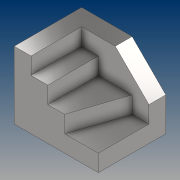
# Autodesk Inventor part: 15
Saved by Autodesk Inventor 2020.2 (Build 242310000, 310)
## iProperties
Created: 2020-09-17
Part Number: 15
Material: 鋼、碳鋼
Document SubType Name: Modeling
Designer: user
Density: 7.85 g/cm^3
Appearance: 半拋光
Mass: 412.125 g
Surface Area: 105.991 cm^2
Volume: 52.5 cm^3
Author: user
Autodesk Inventor part; units mm, degrees
ref_plane "YZ Plane" through (0, 0, 0) normal (1, 0, 0) x (0, 1, 0)
ref_plane "XZ Plane" through (0, 0, 0) normal (0, 1, 0) x (-1, 0, 0)
ref_plane "XY Plane" through (0, 0, 0) normal (0, 0, 1) x (1, 0, 0)
sketch "草圖1" plane through (0, 0, 0) normal (0, 1, 0) x (-1, 0, 0)
  line L0 (0, 0) -> (-50, 0)
  line L1 (-50, 0) -> (-50, -40)
  line L2 (-50, -40) -> (0, -40)
  line L3 (0, -40) -> (0, 0)
  dimension "d0" = 50
  dimension "d1" = 40
  constraints: 8 end point, 2 parallel, 1 horizontal, 1 perpendicular
  measures "d0" distance of L0.start L0.end
  measures "d1" distance of L2.end L0.start
extrude "擠出1" add sketch "草圖1" along normal blind 40
sketch "草圖2" plane through (0, 0, 0) normal (0, 0, 1) x (1, 0, 0)
  line L0 (0, 0) -> (0, 40) projected
  line L1 (0, 40) -> (50, 40) projected
  line L2 (50, 40) -> (50, 0) projected
  line L3 (50, 0) -> (0, 0) projected
  line L4 (0, 40) -> (50, 40) projected
  line L5 (10, 40) -> (10, 30)
  line L6 (10, 30) -> (20, 30)
  line L7 (20, 30) -> (20, 20)
  line L8 (20, 20) -> (40, 20)
  line L9 (40, 20) -> (40, 10)
  line L10 (40, 10) -> (50, 10)
  dimension "d4" = 10
  dimension "d5" = 20
  dimension "d6" = 30
  dimension "d7" = 10
  dimension "d8" = 20
  dimension "d9" = 40
  constraints: 12 end point, 4 perpendicular, 2 point on line, 2 vertical
  measures "d4" distance between parallel lines of L3 L10
  measures "d5" distance between parallel lines of L3 L8
  measures "d6" distance between parallel lines of L3 L6
  measures "d7" distance between parallel lines of L5 L0
  measures "d8" distance between parallel lines of L7 L0
  measures "d9" distance between parallel lines of L9 L0
extrude "擠出2" cut sketch "草圖2" against normal blind 30 contours L1 L2 L10 L9 L8 L7 L6 L5
sketch "草圖3" plane through (0, 0, -30) normal (0, 0, 1) x (1, 0, 0)
  line L0 (10, 40) -> (10, 30) projected
  line L1 (10, 30) -> (20, 30) projected
  line L2 (20, 30) -> (20, 20) projected
  line L3 (20, 20) -> (40, 20) projected
  line L4 (40, 20) -> (40, 10) projected
  line L5 (40, 10) -> (50, 10) projected
  line L6 (50, 40) -> (50, 10) projected
  line L7 (10, 40) -> (50, 40) projected
  line L8 (0, 40) -> (10, 40) projected
  line L9 (0, 0) -> (0, 40) projected
  line L10 (50, 0) -> (0, 0) projected
  line L11 (50, 10) -> (50, 0) projected
  line L12 (30, 40) -> (50, 20)
  dimension "d12" = 20
  dimension "d13" = 20
  constraints: 2 end point, 1 midpoint, 1 point on line
  measures "d12" distance of L6.start L12.start
  measures "d13" distance from line of L7 L12.end
extrude "擠出3" cut sketch "草圖3" against normal blind 10 contours L7 L6 L12
sketch "草圖4" plane through (20, 20, 0) normal (0, 1, 0) x (1, 0, 0)
  line L0 (20, 30) -> (20, 0) projected
  line L1 (20, 0) -> (0, 0) projected
  line L2 (0, 30) -> (0, 0) projected
  line L3 (20, 30) -> (0, 30) projected
  line L4 (30, 30) -> (20, 30) projected
  line L5 (30, 40) -> (30, 30) projected
  line L6 (-20, 40) -> (30, 40) projected
  line L7 (-20, 0) -> (-20, 40) projected
  line L8 (0, 0) -> (-20, 0) projected
  line L9 (10, 0) -> (20, 30)
  line L10 (20, 30) -> (0, 30) projected
  line L11 (30, 30) -> (30, 0) projected
  point P0 (20, 30)
  dimension "d16" = 10
  dimension "d17" = 20
  constraints: 2 end point, 1 midpoint, 1 point on line
  measures "d16" distance from line of L5 L9.end
  measures "d17" distance from line of L11 L9.start
extrude "擠出4" cut sketch "草圖4" against normal up to surface (10 mm away) contours L0 L1 L9
